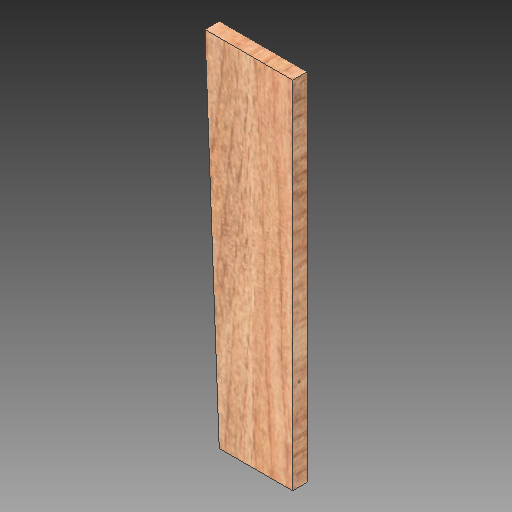
# Autodesk Inventor part: internalSupportTop2
Saved by Autodesk Inventor 2019 (Build 230136000, 136)
## iProperties
Company: FABLAB Torino
Created: 2019-01-11
Part Number: internalSupportTop2
Material: Wood (Birch)
Document SubType Name: Modeling
Designer: Giancarlo
Density: 0.55 g/cm^3
Appearance: Birch - Natural Polished
Description: MultiLayer 10mm
Author: Giancarlo
Title: La Panca - Flower Vase
Subject: Construction MOld
Autodesk Inventor part; units mm, degrees
ref_plane "YZ Plane" through (0, 0, 0) normal (1, 0, 0) x (0, 1, 0)
ref_plane "XZ Plane" through (0, 0, 0) normal (0, 1, 0) x (-1, 0, 0)
ref_plane "Work Plane1" through (0, 0, 0) normal (0, 0, 1) x (1, 0, 0)
sketch "Sketch1" plane through (0, 0, 0) normal (0, 0, 1) x (1, 0, 0)
  line L0 (79.0115, 0) -> (-2.0516, 0) construction
  line L1 (-2.0516, 0) -> (-52.0596, 0) construction
  line L2 (-52.0596, 0) -> (-52.0596, 3) construction
  line L3 (-52.0596, 3) -> (-2.0516, 3) construction
  line L4 (-2.0516, 3) -> (79.0115, 3) construction
  line L5 (79.0115, 3) -> (79.0115, 0) construction
  line L6 (-2.0516, 0) -> (-2.0516, 3) construction
  spline S0 degree 3 poles (-55.0581, -0.1199) (-56.7063, 41.0676) (-58.3545, 82.2551) (-61.6504, 164.6284) (-63.2982, 205.8142) (-64.9459, 247) knots -24.731766 -24.731766 -24.731766 -24.731766 -12.36562 -12.36562 0 0 0 0 construction
  spline S1 degree 3 poles (-64.9459, 247) (-64.6127, 247.0133) (-64.2795, 247.0266) (-63.6132, 247.0533) (-63.28, 247.0666) (-62.9468, 247.0799) knots -0.200064 -0.200064 -0.200064 -0.200064 -0.100032 -0.100032 0 0 0 0 construction
  spline S2 degree 3 poles (-62.9468, 247.0799) (-61.299, 205.8913) (-59.6511, 164.7026) (-56.3552, 82.3293) (-54.7072, 41.1447) (-53.0591, -0.04) knots -24.731955 -24.731955 -24.731955 -24.731955 -12.365476 -12.365476 -0.000192 -0.000192 -0.000192 -0.000192 construction
  spline S3 degree 3 poles (-53.0591, -0.04) (-53.3922, -0.0533) (-53.7254, -0.0666) (-54.3917, -0.0933) (-54.7249, -0.1066) (-55.0581, -0.1199) knots -0.200058 -0.200058 -0.200058 -0.200058 -0.100029 -0.100029 0 0 0 0 construction
  line L7 (-2.0516, 0) -> (-53.0591, -0.04)
  line L8 (-62.9468, 247.0799) -> (-2.0516, 247.0799)
  line L9 (-2.0516, 247.0799) -> (-2.0516, 0)
  line L10 (-53.0591, -0.04) -> (-62.9468, 247.0799)
  constraints: 22 end point, 4 horizontal, 3 vertical, 2 perpendicular, 22 other
extrude "Extrusion1" add sketch "Sketch1" along normal blind 10
body "Solid1"
